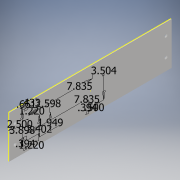
# Autodesk Inventor part: nmt_sidepanel_20in
Saved by Autodesk Inventor 2017 (Build 210142000, 142)
## iProperties
Created: 2017-02-19
Part Number: nmt_sidepanel_20in
Material: Generic
Document SubType Name: Modeling
Designer: Zara
Density: 1 g/cm^3
Appearance: Default
Author: Zara
Autodesk Inventor part; units mm, degrees
ref_plane "YZ Plane" through (0, 0, 0) normal (1, 0, 0) x (0, 1, 0)
ref_plane "XZ Plane" through (0, 0, 0) normal (0, 1, 0) x (-1, 0, 0)
ref_plane "XY Plane" through (0, 0, 0) normal (0, 0, 1) x (1, 0, 0)
sketch "Sketch1" plane through (0, 0, 0) normal (1, 0, 0) x (0, 1, 0)
  line L0 (-66.294, 254) -> (66.294, 254)
  line L1 (66.294, 254) -> (66.294, -254)
  line L2 (66.294, -254) -> (-66.294, -254)
  line L3 (-66.294, -254) -> (-66.294, 254)
  line L4 (-66.294, 254) -> (66.294, -254) construction
  line L5 (66.294, 254) -> (-66.294, -254) construction
  point P0 (0, 0)
  dimension "d0" = 508
  dimension "d1" = 132.588
  constraints: 12 end point, 2 midpoint, 2 parallel, 1 horizontal, 1 perpendicular
  measures "d0" distance of L0.end L1.end
  measures "d1" distance of L1.end L2.end
extrude "pdu nmt right side panel" add sketch "Sketch1" along normal blind 3.175
sketch "snap psu" plane through (0, 0, 0) normal (-1, 0, 0) x (0, 0, 1)
  line L0 (-21.209, -49.5046) -> (-21.209, 49.5046) construction
  line L1 (-21.209, 49.5046) -> (190.5, 49.5046) construction
  line L2 (190.5, 49.5046) -> (190.5, -49.5046) construction
  line L3 (190.5, -49.5046) -> (-21.209, -49.5046) construction
  line L4 (179.5018, -49.5046) -> (179.5018, 49.5046) construction
  line L5 (-254, 66.294) -> (254, 66.294) projected
  line L6 (254, -66.294) -> (254, 66.294) projected
  line L7 (159.512, 11.5062) -> (159.512, -19.2811) construction
  line L8 (-8.509, 39.497) -> (-8.509, -39.497) construction
  line L9 (124.5108, 0) -> (186.1095, 0) construction
  point P0 (0, 0)
  point P1 (159.512, -39.497)
  dimension "d19" = 10.0076
  dimension "d20" = 30.988
  dimension "d21" = 99.0092
  dimension "d22" = 12.7
  dimension "d23" = 10.9982
  dimension "d24" = 16.7894
  dimension "d25" = 63.5
  dimension "d33" = 10.0076
  dimension "d34" = 89.0016
  dimension "d35" = 30.988
  dimension "d36" = 61.0108
  dimension "d37" = 65.9892
  dimension "d38" = 49.5046
  dimension "d39" = 199.009
  dimension "d40" = 199.009
  constraints: 16 end point, 2 parallel, 2 perpendicular, 2 point on line, 1 horizontal, 1 vertical
  measures "d19" distance from line of L3 point (159.512, -39.497)
  measures "d20" distance from line of point (159.512, -39.497) L2
  measures "d21" distance of L1.end L2.end
  measures "d22" distance from line of L0 L8.end
  measures "d23" distance between parallel lines of L4 L2
  measures "d24" distance between parallel lines of L5 L1
  measures "d25" distance between parallel lines of L2 L6
  measures "d33" distance from line of L8.end L3
  measures "d34" distance from line of L8.start L3
  measures "d35" distance from line of L7.start L2
  measures "d36" distance from line of L7.start L3
  measures "d37" distance from line of L9.start L2
  measures "d38" distance from line of L9.start L3
  measures "d39" distance from line of L8.end L2
  measures "d40" distance from line of L8.start L2
sketch "Sketch5" plane through (3.175, 0, 0) normal (1, 0, 0) x (0, 0, -1)
  point P0 (0, 0)
  point P1 (8.509, 39.497)
  point P2 (8.509, -39.497)
  point P3 (-124.5108, 0)
  point P4 (-159.512, 11.5062)
  point P5 (-159.512, -39.497)
hole "snap psu holes" at (3.175, 11.5062, 159.512) at (3.175, -39.497, 159.512) at (3.175, 0, 124.5108) at (3.175, 39.497, -8.509) at (3.175, -39.497, -8.509) direction (-1, 0, 0) diameter 3.4036 end through all clearance for "Countersunk Flat Head Screw ISO 2009/7046" size "M3" standard "ISO"
sketch "brackets" plane through (3.175, 0, 0) normal (1, 0, 0) x (0, 0, -1)
  line L0 (-254, 66.294) -> (-254, -66.294) construction
  line L1 (-249.428, 54.61) -> (-230.378, 54.61) construction
  line L2 (-230.378, 54.61) -> (-230.378, -54.61) construction
  line L3 (-230.378, -54.61) -> (-249.428, -54.61) construction
  line L4 (-249.428, -54.61) -> (-249.428, 54.61) construction
  line L5 (254, 66.294) -> (-254, 66.294) construction
  line L6 (254, -66.294) -> (254, 66.294) construction
  line L7 (249.428, 54.61) -> (230.378, 54.61) construction
  line L8 (230.378, 54.61) -> (230.378, -54.61) construction
  line L9 (230.378, -54.61) -> (249.428, -54.61) construction
  line L10 (249.428, -54.61) -> (249.428, 54.61) construction
  point P0 (0, 0)
  point P1 (236.3724, 29.21)
  point P2 (236.3724, -29.21)
  point P3 (-236.3724, 29.21)
  point P4 (-236.3724, -29.21)
  dimension "d38" = 49.5046
  dimension "d41" = 11.684
  dimension "d42" = 109.22
  dimension "d43" = 19.05
  dimension "d44" = 11.684
  dimension "d45" = 19.05
  dimension "d46" = 109.22
  dimension "d47" = 25.4
  dimension "d48" = 5.9944
  dimension "d49" = 25.4
  dimension "d50" = 5.9944
  dimension "d51" = 25.4
  dimension "d53" = 25.4
  dimension "d54" = 5.9944
  dimension "d55" = 5.9944
  dimension "d70" = 4.572
  dimension "d71" = 4.572
  constraints: 18 end point, 4 parallel, 2 horizontal, 2 perpendicular
  measures "d41" distance between parallel lines of L5 L1
  measures "d42" distance of L1.end L2.end
  measures "d43" distance of L1.start L1.end
  measures "d44" distance between parallel lines of L7 L5
  measures "d45" distance of L7.start L7.end
  measures "d46" distance of L7.end L8.end
  measures "d47" distance from line of L1 point (-236.372, 29.21)
  measures "d48" distance from line of L2 point (-236.372, 29.21)
  measures "d49" distance from line of point (-236.372, -29.21) L3
  measures "d50" distance from line of L2 point (-236.372, -29.21)
  measures "d51" distance from line of L7 point (236.372, 29.21)
  measures "d53" distance from line of point (236.372, -29.21) L9
  measures "d54" distance from line of L8 point (236.372, -29.21)
  measures "d55" distance from line of L8 point (236.372, 29.21)
  measures "d70" distance between parallel lines of L0 L4
  measures "d71" distance between parallel lines of L10 L6
hole "Hole4" at (3.175, 29.21, -236.3724) at (3.175, -29.21, -236.3724) at (3.175, -29.21, 236.3724) at (3.175, 29.21, 236.3724) direction (-1, 0, 0) diameter 4.2926 end through all countersink diameter 9.398 countersink angle 90 clearance for "Countersunk Flat Head Screw ISO 2009/7046" size "M4" standard "ISO"
body "Solid1"
